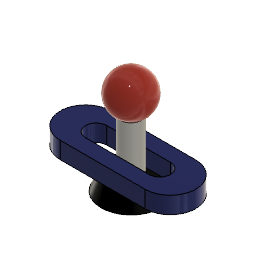
Joystick (Autodesk Fusion 360 design; units mm, degrees)
part number: 2026-07-03-15-09-44-805
part number: 2026-07-03-15-25-33-935
Autodesk Fusion 360 part; units mm, degrees
sketch "草图1" plane through (0, 0, 0) normal (0, 0, 1) x (1, 0, 0)
  line L0 (0, 30) -> (-100, 30)
  arc A0 (-100, 30) -> (-100, -30) centre (-100, 0) ccw
  line L1 (-100, -30) -> (0, -30)
  arc A1 (0, -30) -> (0, 30) centre (0, 0) ccw
  line L2 (0, 0) -> (-100, 0) construction
  dimension "d1" = 60
  constraint tangent L0 A0
  constraint tangent A0 L1
  constraint parallel L0 L1
  constraint tangent L1 A1
  constraint tangent L0 A1
  constraint horizontal L2
  constraint coincident A1.centre L2.start
  measures "d1" diameter of A0
extrude "拉伸1" add sketch "草图1" along normal blind 20 makes body 1
sketch "草图2" plane through (0, 0, 20) normal (0, 0, 1) x (-1, 0, 0)
  arc A0 (0, 30) -> (0, -30) centre (0, 0) ccw
  line L0 (0, -30) -> (100, -30)
  arc A1 (100, -30) -> (100, 30) centre (100, 0) ccw
  line L1 (100, 30) -> (0, 30)
  line L2 (12.5, -12.5) -> (87.5, -12.5)
  arc A2 (87.5, -12.5) -> (87.5, 12.5) centre (87.5, 0) ccw
  line L3 (87.5, 12.5) -> (12.5, 12.5)
  arc A3 (12.5, 12.5) -> (12.5, -12.5) centre (12.5, 0) ccw
  line L4 (0, 0) -> (100, 0) construction
  dimension "d4" = 25
  constraint tangent L2 A2
  constraint tangent A2 L3
  constraint parallel L2 L3
  constraint tangent L3 A3
  constraint tangent L2 A3
  constraint coincident A3 A0.centre
  constraint coincident A2 A1.centre
  constraint coincident A2.centre L4
  constraint coincident A3.centre L4
  constraint coincident A1.centre L4.end
  constraint horizontal L4
  constraint coincident A0.centre L4.start
  measures "d4" diameter of A2
extrude "拉伸2" cut sketch "草图2" along normal through all and the other way through all contours L2 A2 L3 A3 bodies 1
sketch "草图3" plane through (0, 0, 0) normal (0, 0, 1) x (1, 0, 0)
  circle A0 centre (107.4857, 14.9164) radius 35
  dimension "d7" = 70
  measures "d7" diameter of A0
extrude "拉伸1'" add sketch "草图3" along normal blind 20 draft -20 separate body makes body 2 in component "handle"
sketch "草图4" plane through (0, 0, 20) normal (0, 0, 1) x (-1, 0, 0)
  circle A0 centre (-107.4857, -14.9164) radius 27.7206
  circle A1 centre (-107.4857, -14.9164) radius 12.5
  dimension "d10" = 25
  constraint concentric A0 A1
  measures "d10" diameter of A1
extrude "拉伸2'" add sketch "草图4" along normal blind 80 contours A1 bodies 2 in component "handle"
sphere "球体基本要素1" add diameter 50 placed x (-1, 0, 0) y (0, -1, 0) z (0, 0, 1) at (107.4857, 14.9164, 100) bodies 2 in component "handle"
component "handle" placed x (1, 0, 0) y (0, 1, 0) z (0, 0, 1) at (-119.4857, -14.9164, -20)
